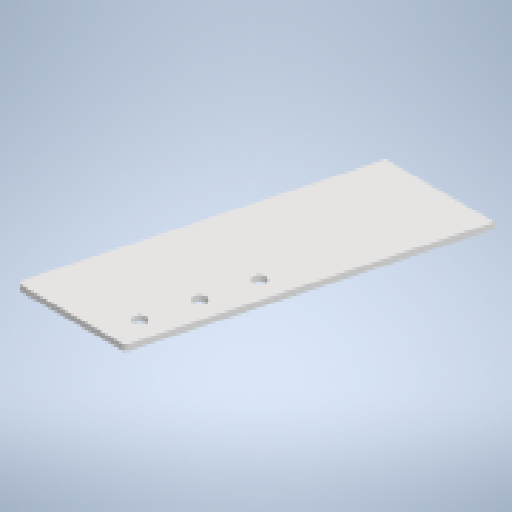
# Autodesk Inventor part: держатель полки 1
Saved by Autodesk Inventor 2024.2 (Build 282272000, 272)
## iProperties
Created: 2024-06-15
Part Number: держатель полки 1
Material: Generic
Document SubType Name: Sheet Metal
Designer: admin
Density: 1 g/cm^3
Sheet Metal Rule: Default
Appearance: Default
Author: admin
Autodesk Inventor part; units mm, degrees
ref_plane "YZ Plane" through (0, 0, 0) normal (1, 0, 0) x (0, 1, 0)
ref_plane "XZ Plane" through (0, 0, 0) normal (0, 1, 0) x (-1, 0, 0)
ref_plane "XY Plane" through (0, 0, 0) normal (0, 0, 1) x (1, 0, 0)
sketch "Sketch1" plane through (0, 0, 0) normal (0, 0, 1) x (1, 0, 0)
  line L0 (-160, 0) -> (160, 0)
  line L1 (160, 0) -> (160, -200) construction
  line L2 (160, -200) -> (-160, -200)
  line L3 (-160, -200) -> (-160, 0) construction
  line L4 (-160, 0) -> (-213.5898, -200)
  line L5 (-213.5898, -200) -> (-160, -200)
  line L6 (160, 0) -> (213.5898, -200)
  line L7 (213.5898, -200) -> (160, -200)
  line L8 (0, 0) -> (-53.5898, -200)
  line L9 (-160, 0) -> (-93.0127, 250)
  line L10 (-93.0127, 250) -> (66.9873, 250)
  line L11 (66.9873, 250) -> (0, 0)
  line L12 (14.7372, 55) -> (74.7372, 55)
  line L13 (74.7372, 55) -> (74.7372, 250)
  line L14 (74.7372, 250) -> (66.9873, 250)
  dimension "d1" = 200
  dimension "d2" = 15
  dimension "d29" = 160
  dimension "d37" = 255
  dimension "d38" = 195
  dimension "d39" = 60
  measures "d1" distance of L0.end L1.end
  measures "d2" angle of L3 L4
  measures "d29" distance of L8.end L4.end
  measures "d37" distance between parallel lines of L2 L12
  measures "d38" distance between parallel lines of L10 L12
  measures "d39" distance from line of L12.start L13
extrude "Plate1" add sketch "Sketch1" along normal blind 8 contours L9 L10 L11 L0 | L0 L8 L2 L5 L4 | L11 L14 L13 L12
sketch "Sketch3" plane through (0, 0, 8) normal (0, 0, 1) x (1, 0, 0)
  line L0 (-38.9896, -29.6) -> (-73.9302, -160) construction
  line L1 (-213.5898, -200) -> (-93.0127, 250) projected
  line L2 (51.0104, 209.2028) -> (51.0104, 79.2815) construction
  point P0 (0, 0)
  point P1 (-56.4599, -94.8)
  point P2 (-150, 0)
  point P3 (-93.0127, 250)
  point P4 (-19.4263, -72.5)
  dimension "d28" = 135
  dimension "d36" = 90
  constraints: 4 end point, 2 coincident, 1 midpoint, 1 vertical, 2 other
  measures "d28" distance of L0.start L0.end
  measures "d36" distance from line of point (-38.99, -29.6) L2
hole "Hole1" at (-38.9896, -29.6, 8) at (-56.4599, -94.8, 8) at (-73.9302, -160, 8) at (51.0104, 209.2028, 8) at (51.0104, 79.2815, 8) direction (0, 0, -1) diameter 17 end through all
fillet "Corner Round1" radius 6 2 edges at (-213.5898, -200, 4) (-53.5898, -200, 4)
sketch "Sketch5" plane through (0, 0, 0) normal (0, 0, -1) x (-1, 0, 0)
  circle A0 centre (73.9302, -160) radius 8.5 projected
  circle A1 centre (56.4599, -94.8) radius 8.5 projected
  circle A2 centre (38.9896, -29.6) radius 8.5 projected
  arc A3 (52.3982, -195.5529) -> (58.1938, -200) centre (58.1938, -194) ccw projected
  line L0 (205.7705, -200) -> (58.1938, -200) projected
  arc A4 (205.7705, -200) -> (211.566, -192.4471) centre (205.7705, -194) ccw projected
  line L1 (93.0127, 250) -> (211.566, -192.4471) projected
  line L2 (-74.7372, 250) -> (93.0127, 250) projected
  line L3 (-74.7372, 55) -> (-74.7372, 250) projected
  line L4 (-14.7372, 55) -> (-74.7372, 55) projected
  line L5 (52.3982, -195.5529) -> (-14.7372, 55) projected
  line L6 (-74.7372, 236) -> (-29.7372, 242.3243)
  line L7 (-29.7372, 242.3243) -> (-29.7372, 250)
  point P0 (0, 0)
  dimension "d30" = 14
  dimension "d31" = 45
  dimension "d32" = 98
  constraints: 4 end point, 2 point on line, 1 vertical
  measures "d30" distance from line of L6.start L2
  measures "d31" distance between parallel lines of L3 L7
  measures "d32" angle of L3 L6
extrude "Extrusion1" cut sketch "Sketch5" against normal through all contours L3 L2 L7 L6
fillet "Fillet1" radius 2 2 edges at (74.7372, 236, 4) (29.7372, 242.3243, 4)
equation "\"d9\" = Thickness"
equation "\"d3\" = Thickness"
equation "\"BendRadius\" = Thickness"
equation "\"BendReliefWidth\" = Thickness"
equation "\"BendReliefDepth\" = 0.5 * Thickness"
equation "\"CornerReliefSize\" = 4 * Thickness"
equation "\"MinimumRemnant\" = 2 * Thickness"
equation "\"TransitionRadius\" = BendRadius"
equation "\"JacobiRadiusSize\" = BendRadius"
equation "\"GapSize\" = Thickness"
equation "\"Thickness\" = 8"
body "Solid1"
